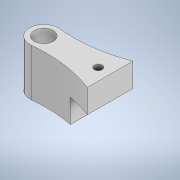
# Autodesk Inventor part: stability copy2
Saved by Autodesk Inventor 2020 (Build 240168000, 168)
## iProperties
Created: 2019-07-11
Part Number: stability copy2
Material: Generic
Document SubType Name: Modeling
Designer: ColinP
Density: 1 g/cm^3
Appearance: Default
Mass: 5.85901 g
Surface Area: 26.8401 cm^2
Volume: 5.85901 cm^3
Author: ColinP
Autodesk Inventor part; units mm, degrees
ref_plane "YZ Plane" through (0, 0, 0) normal (1, 0, 0) x (0, 1, 0)
ref_plane "XZ Plane" through (0, 0, 0) normal (0, 1, 0) x (-1, 0, 0)
ref_plane "XY Plane" through (0, 0, 0) normal (0, 0, 1) x (1, 0, 0)
sketch "Sketch1" plane through (0, 0, 0) normal (0, 1, 0) x (-1, 0, 0)
  line L0 (0, 0) -> (28.575, 0)
  line L1 (28.575, 0) -> (0, 0)
  line L2 (0, 0) -> (-14.2875, -24.7467)
  line L3 (0, 0) -> (28.575, 0) construction
  line L4 (0, 0) -> (-14.2875, 24.7467)
  line L5 (0, 0) -> (28.575, 0) construction
  circle A0 centre (28.575, 0) radius 2.54
  circle A1 centre (-14.2875, -24.7467) radius 2.54
  circle A2 centre (-14.2875, 24.7467) radius 2.54
  circle A3 centre (0, 0) radius 3.175
  circle A4 centre (0, 0) radius 6.35
  line L6 (-1.5875, -2.7496) -> (0, 0)
  line L7 (0, 0) -> (-6.35, 0)
  circle A5 centre (-14.2875, 24.7467) radius 3.81
  circle A6 centre (28.575, 0) radius 3.81
  circle A7 centre (-14.2875, -24.7467) radius 3.81
  line L8 (30.6811, 3.175) -> (-12.1814, 27.9217)
  line L9 (28.2054, -3.792) -> (-10.8187, -26.3226)
  line L10 (-18.0975, 24.7467) -> (-18.0975, -24.7467)
  line L11 (0, 0) -> (5.0525, -8.8146)
  line L12 (0, 0) -> (5.1463, 8.7602)
  line L13 (0, 0) -> (-10.16, 0)
  arc A8 (28.2054, -3.792) -> (-10.8187, -26.3226) centre (24.4473, -42.344) ccw
  arc A9 (-10.8187, 26.3226) -> (28.2054, 3.792) centre (24.4473, 42.344) ccw
  arc A10 (-17.3867, -22.5305) -> (-17.3867, 22.5305) centre (-48.8947, 0) ccw
  point P0 (5.1074, 8.7829)
  point P1 (-10.16, 0.0317)
  point P2 (30.2716, 3.4114)
  point P3 (28.2054, 3.792)
  point P4 (-10.8187, 26.3226)
  point P5 (-17.3867, 22.5305)
  point P6 (-17.3867, -22.5305)
  dimension "d9" = 6.35
  dimension "d41" = 12.7
  dimension "d0" = 28.575
  dimension "d1" = 28.575
  dimension "d2" = 120
  dimension "d3" = 28.575
  dimension "d4" = 120
  dimension "d5" = 5.08
  dimension "d6" = 5.08
  dimension "d7" = 5.08
  dimension "d42" = 7.62
  dimension "d43" = 7.62
  dimension "d44" = 7.62
  dimension "d47" = 10.16
  dimension "d48" = 10.16
  dimension "d49" = 10.16
  dimension "d52" = 360
  constraints: 28 end point, 15 point on circle, 9 centre point, 8 coincident, 4 horizontal, 3 tangent, 2 collinear, 2 equal length, 2 point on line, 1 horizontal alignment, 21 other
  measures "d0" distance of L0.start L0.end
  measures "d1" distance of L0.start L2.end
  measures "d2" angle of L2 L3
  measures "d3" distance of L0.start L4.end
  measures "d4" angle of L5 L4
  measures "d5" diameter of A0
  measures "d6" diameter of A1
  measures "d7" diameter of A2
  measures "d42" diameter of A5
  measures "d43" diameter of A6
  measures "d44" diameter of A7
  measures "d47" distance of L6.end L11.end
  measures "d48" distance of L6.end L12.end
  measures "d49" distance of L6.end L13.end
extrude "Extrusion4" add sketch "Sketch1" along normal blind 12.7 contours A3 L12 A4 L0 | L0 A4 L11 A3 | A3 L11 A4 L2 | L2 A4 L7 A3 | A3 L7 A4 L4 | L4 A4 L12 A3 | A4 L12 A9 A6 L0 | L0 A6 A8 L11 A4 | A4 L11 A8 A7 L2 | L2 A7 A10 L13 A4 | A4 L13 A10 A5 L4 | L4 A5 A9 L12 A4 | A6 L8 | A7 | A5 picked at (31.8987, 0.5122)
sketch "Sketch21" plane through (0, 12.7, 0) normal (0, 1, 0) x (1, 0, 0)
  circle A0 centre (-28.575, 0) radius 2.54 projected
  arc A1 (-28.2054, 3.792) -> (10.8187, 26.3226) centre (-24.4473, 42.344) ccw projected
  arc A2 (10.8187, -26.3226) -> (-28.2054, -3.792) centre (-24.4473, -42.344) ccw projected
  arc A3 (-28.2054, 3.792) -> (10.8187, 26.3226) centre (-24.4473, 42.344) ccw projected
  arc A4 (-28.2054, 3.792) -> (-30.6811, -3.175) centre (-28.575, 0) ccw projected
  line L0 (-30.6811, -3.175) -> (-30.2716, -3.4114) projected
  arc A5 (-30.2716, -3.4114) -> (-28.2054, -3.792) centre (-28.575, 0) ccw projected
  arc A6 (10.8187, -26.3226) -> (-28.2054, -3.792) centre (-24.4473, -42.344) ccw projected
  arc A7 (10.8187, -26.3226) -> (17.3867, -22.5305) centre (14.2875, -24.7467) ccw projected
  arc A8 (17.3867, 22.5305) -> (17.3867, -22.5305) centre (48.8947, 0) ccw projected
  arc A9 (17.3867, 22.5305) -> (10.8187, 26.3226) centre (14.2875, 24.7467) ccw projected
  circle A10 centre (-28.575, 0) radius 2.54 projected
  circle A11 centre (0, 0) radius 3.175 projected
  circle A12 centre (14.2875, -24.7467) radius 2.54 projected
  circle A13 centre (14.2875, 24.7467) radius 2.54 projected
  line L1 (0, 0) -> (-13.6784, 0)
  line L2 (-13.6784, 0) -> (-28.575, 0)
  line L3 (0, 0) -> (-10.795, 0)
  line L4 (-10.795, 0) -> (-10.795, 6.095)
  arc A14 (-28.2054, 3.792) -> (10.8187, 26.3226) centre (-24.4473, 42.344) ccw projected
  line L5 (-10.795, 0) -> (-10.795, -6.095)
  point P0 (10.8187, -26.3226)
  point P1 (10.8187, 26.3226)
  dimension "d107" = 10.795
  constraints: 10 end point, 2 point on circle, 2 point on line, 1 collinear, 1 horizontal, 1 perpendicular
  measures "d107" distance of L1.start L3.end
sketch "Sketch22" plane through (0, 0, 0) normal (0, -1, 0) x (1, 0, 0)
  line L0 (0, 0) -> (-17.145, 0)
  line L1 (-17.145, 0) -> (-17.145, -4.3038)
  arc A0 (10.8187, -26.3226) -> (-28.2054, -3.792) centre (-24.4473, -42.344) ccw projected
  line L2 (-17.145, 0) -> (-17.145, 4.3038)
  arc A1 (-28.2054, 3.792) -> (10.8187, 26.3226) centre (-24.4473, 42.344) ccw projected
  arc A2 (10.8187, -26.3226) -> (-28.2054, -3.792) centre (-24.4473, -42.344) ccw projected
  arc A3 (10.8187, -26.3226) -> (17.3867, -22.5305) centre (14.2875, -24.7467) ccw projected
  arc A4 (17.3867, 22.5305) -> (17.3867, -22.5305) centre (48.8947, 0) ccw projected
  arc A5 (17.3867, 22.5305) -> (10.8187, 26.3226) centre (14.2875, 24.7467) ccw projected
  arc A6 (-28.2054, 3.792) -> (10.8187, 26.3226) centre (-24.4473, 42.344) ccw projected
  arc A7 (-28.2054, 3.792) -> (-30.2716, 3.4114) centre (-28.575, 0) ccw projected
  line L3 (-30.6811, 3.175) -> (-30.2716, 3.4114) projected
  arc A8 (-30.6811, 3.175) -> (-28.2054, -3.792) centre (-28.575, 0) ccw projected
  circle A9 centre (-28.575, 0) radius 2.54 projected
  circle A10 centre (0, 0) radius 3.175 projected
  circle A11 centre (14.2875, 24.7467) radius 2.54 projected
  circle A12 centre (14.2875, -24.7467) radius 2.54 projected
  point P0 (10.8187, -26.3226)
  point P1 (10.8187, 26.3226)
  dimension "d108" = 17.145
  constraints: 6 end point, 2 point on circle, 1 horizontal, 1 perpendicular, 1 point on line
  measures "d108" distance of L0.start L0.end
extrude "Extrusion10" cut sketch "Sketch22" against normal blind 6.35 contours L2 A1 A5 A4 A3 A0 L1
extrude "Extrusion11" cut sketch "Sketch21" against normal blind 6.35 contours A1 A9 A8 A7 A2 L5 L4
sketch "Sketch23" plane through (0, 12.7, 0) normal (0, 1, 0) x (1, 0, 0)
  point P0 (0, 0)
sketch "Sketch24" plane through (0, 6.35, 0) normal (0, -1, 0) x (1, 0, 0)
  line L0 (-17.145, -4.3038) -> (-17.145, 4.3038) projected
  line L1 (-17.145, 0) -> (-10.795, 0)
  line L2 (-10.795, -6.095) -> (-10.795, 6.095) projected
  line L3 (-13.97, 0) -> (-13.97, 5.0532)
  arc A0 (-17.145, 4.3038) -> (-10.795, 6.095) centre (-24.4473, 42.344) ccw projected
  line L4 (-13.97, 0) -> (-13.97, -5.0532)
  arc A1 (-10.795, -6.095) -> (-17.145, -4.3038) centre (-24.4473, -42.344) ccw projected
  point P0 (0, 0)
  constraints: 6 end point, 3 midpoint, 2 point on circle, 1 perpendicular, 1 point on line
hole "Hole8" at (-13.97, 6.35, 0) direction (0, 1, 0) diameter 2.1129 depth 7.7978 thread size "M2.6x0.45" class "6H" standard "ISO Metric profile"
body "Solid3"
